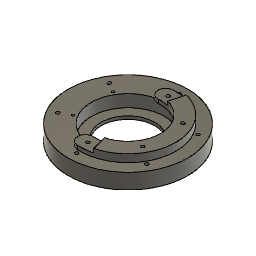
mounting_flange (Autodesk Fusion 360 design; units mm, degrees)
Autodesk Fusion 360 part; units mm, degrees
sketch "Sketch1" plane through (0, 0, 0) normal (0, 1, 0) x (1, 0, 0)
  circle A0 centre (0, 0) radius 56 construction
  circle A1 centre (0, 0) radius 78
  circle A2 centre (0, 0) radius 67 construction
  circle A3 centre (0, 67) radius 2.25
  circle A4 centre (-58.0237, 33.5) radius 2.25
  circle A5 centre (-58.0237, -33.5) radius 2.25
  circle A6 centre (0, -67) radius 2.25
  circle A7 centre (58.0237, -33.5) radius 2.25
  circle A8 centre (58.0237, 33.5) radius 2.25
  circle A9 centre (0, 0) radius 35
  circle A10 centre (0, 0) radius 63.2009
  circle A11 centre (0, 0) radius 59.2009
  dimension "d1" = 156
  dimension "d2" = 112
  dimension "d3" = 134
  dimension "d4" = 4.5
  dimension "d6" = 360
  dimension "d7" = 70
  dimension "d8" = 4
  constraint coincident A0.centre A1.centre
  constraint concentric A0 A1
  constraint concentric A1 A2
  constraint coincident A2 A3.centre
  constraint vertical A0.centre A3.centre
  constraint concentric A0 A9
  constraint concentric A0 A10
  constraint concentric A1 A11
  measures "d1" diameter of A1
  measures "d2" diameter of A0
  measures "d3" diameter of A2
  measures "d4" diameter of A3
  measures "d7" diameter of A9
  measures "d8" distance of A10 A11
extrude "Extrude1" add sketch "Sketch1" along normal blind 20 contours A1 | A10 | A11 makes body 1
extrude "Extrude2" cut sketch "Sketch1" along normal blind 2 contours A10 bodies 1
sketch "Sketch2" plane through (0, 20, 0) normal (0, 1, 0) x (-1, 0, 0)
  circle A0 centre (-58.0237, -33.5) radius 2.25
  circle A1 centre (0, 0) radius 35
  circle A2 centre (58.0237, 33.5) radius 2.25
  circle A3 centre (0, 67) radius 2.25
  circle A4 centre (58.0237, -33.5) radius 2.25
  circle A5 centre (-58.0237, 33.5) radius 2.25
  circle A6 centre (0, -67) radius 2.25
  circle A7 centre (0, 0) radius 78
  circle A8 centre (0, 0) radius 47.5 construction
  circle A9 centre (0, 0) radius 62.5
  circle A10 centre (0, 0) radius 48
  circle A11 centre (0, 0) radius 52.5 construction
  circle A12 centre (0, -52.5) radius 1.65
  circle A13 centre (0, -67) radius 2.25
  circle A14 centre (45.4663, -26.25) radius 1.65
  circle A15 centre (45.4663, 26.25) radius 1.65
  circle A16 centre (0, 52.5) radius 1.65
  circle A17 centre (-45.4663, 26.25) radius 1.65
  circle A18 centre (-45.4663, -26.25) radius 1.65
  line L0 (15.6914, -60.4982) -> (10.6701, -41.1388)
  line L1 (-10.6701, 41.1388) -> (-15.6914, 60.4982)
  circle A19 centre (0, 0) radius 42.5
  line L2 (-15.6914, -60.4982) -> (-10.6701, -41.1388)
  line L3 (10.6701, 41.1388) -> (15.6914, 60.4982)
  line L4 (0, 0) -> (0, -19.0746) construction
  circle A20 centre (0, -52.5) radius 2.25
  circle A21 centre (45.4663, -26.25) radius 2.25
  circle A22 centre (45.4663, 26.25) radius 2.25
  circle A23 centre (0, 52.5) radius 2.25
  circle A24 centre (-45.4663, 26.25) radius 2.25
  circle A25 centre (-45.4663, -26.25) radius 2.25
  dimension "d14" = 95
  dimension "d15" = 96
  dimension "d16" = 15
  dimension "d19" = 360
  dimension "d20" = 85
  dimension "d40" = 10
  dimension "d45" = 3.3
  dimension "d46" = 4.5
  dimension "d48" = 360
  constraint concentric A1 A8
  constraint concentric A8 A9
  constraint concentric A9 A10
  constraint concentric A10 A11
  constraint coincident A11 A12.centre
  constraint vertical A1.centre A12.centre
  constraint coincident A9 L0.start
  constraint coincident A9 L1.end
  constraint coincident A1.centre L0
  constraint collinear L0 L1
  constraint concentric A9 A19
  constraint coincident A19 L0.end
  constraint coincident A19 L1.start
  constraint coincident A9 L2.start
  constraint coincident A9 L3.end
  constraint coincident A1.centre L2
  constraint collinear L2 L3
  constraint coincident A19 L2.end
  constraint coincident A19 L3.start
  constraint coincident A1.centre A7.centre
  constraint vertical L4
  constraint symmetric L0.start L2.start L4
  constraint concentric A12 A20
  measures "d14" diameter of A8
  measures "d15" diameter of A10
  measures "d16" distance of A8 A9
  measures "d20" diameter of A19
  measures "d40" distance of A9 A11
  measures "d45" diameter of A12
  measures "d46" diameter of A20
extrude "Extrude7" cut sketch "Sketch2" against normal blind 16 contours A10 L1 A19 L3 | A10 L0 A19 L3 | A10 L0 A19 L2 | A10 L1 A19 L2 | A19 bodies 1
extrude "Extrude8" add sketch "Sketch2" along normal blind 10 separate body contours A9 A10 L1 L3 | A9 A10 L0 L2 | A9 A10 L1 L2 | A10 L1 A19 L3 | A10 L0 A19 L2 | A10 L1 A19 L2 makes body 2
extrude "Extrude10" cut sketch "Sketch2" against normal blind 5 from surface at 10 contours A9 A10 L1 L3 | A9 A10 L0 L2 | A10 L1 A19 L3 | A10 L0 A19 L2 | A20 | A23 bodies 2
fillet "Fillet1" radius 10 4 edges at (-15.6914, 22.5, -60.4982) (-10.6701, 22.5, -41.1388) (-10.6701, 25, 41.1388) (-15.6914, 25, 60.4982) on bodies 2
extrude "Extrude11" cut sketch "Sketch2" against normal blind 15 contours A12 | A14 | A15 | A16 | A17 | A18 bodies 1
